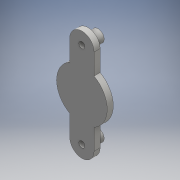
# Autodesk Inventor part: Coperchio Superiore
Saved by Autodesk Inventor 2016 (Build 200138000, 138)
## iProperties
Created: 2016-09-08
Part Number: Coperchio Superiore
Material: Generic
Document SubType Name: Modeling
Designer: Muhammad
Density: 1 g/cm^3
Appearance: Default
Author: Muhammad
Autodesk Inventor part; units mm, degrees
ref_plane "YZ Plane" through (0, 0, 0) normal (1, 0, 0) x (0, 1, 0)
ref_plane "XZ Plane" through (0, 0, 0) normal (0, 1, 0) x (-1, 0, 0)
ref_plane "XY Plane" through (0, 0, 0) normal (0, 0, 1) x (1, 0, 0)
sketch "Sketch1" plane through (0, 0, 0) normal (0, 1, 0) x (-1, 0, 0)
  arc A0 (12, 42.5) -> (-12, 42.5) centre (0, 42.5) ccw
  arc A1 (-12, -42.5) -> (12, -42.5) centre (0, -42.5) ccw
  line L0 (0, 42.5) -> (12, 42.5) construction
  line L1 (0, -42.5) -> (12, -42.5) construction
  line L2 (0, -42.5) -> (-12, -42.5) construction
  line L3 (0, 42.5) -> (-12, 42.5) construction
  line L4 (12, 42.5) -> (12, 21.9317)
  line L5 (12, -42.5) -> (12, -21.9317)
  line L6 (-12, -42.5) -> (-12, -21.9317)
  line L7 (-12, 42.5) -> (-12, 21.9317)
  arc A2 (-12, 21.9317) -> (-12, -21.9317) centre (0, 0) ccw
  arc A3 (12, -21.9317) -> (12, 21.9317) centre (0, 0) ccw
  constraints: 16 end point, 8 point on circle, 4 centre point, 4 point on line, 2 parallel, 1 horizontal, 1 perpendicular, 1 tangent
extrude "Extrusion1" add sketch "Sketch1" along normal blind 6
sketch "Sketch2" plane through (0, 6, 0) normal (0, 1, 0) x (1, 0, 0)
  circle A0 centre (0, 0) radius 10
  circle A1 centre (0, 0) radius 19.5 construction
  arc A2 (-12, -42.5) -> (12, -42.5) centre (0, -42.5) ccw construction
  line L0 (0, -42.5) -> (0, -54.5) construction
  arc A3 (12, 42.5) -> (-12, 42.5) centre (0, 42.5) ccw construction
  line L1 (0, 42.5) -> (0, 54.5) construction
  circle A4 centre (0, -42.5) radius 6
  circle A5 centre (0, -42.5) radius 3
  circle A6 centre (0, 42.5) radius 6
  circle A7 centre (0, 42.5) radius 3
  dimension "d11" = 20
  dimension "d12" = 39
  constraints: 6 centre point, 6 coincident, 4 end point, 2 point on circle, 1 point on line, 1 vertical
  measures "d11" diameter of A0
  measures "d12" diameter of A1
extrude "Extrusion2" add sketch "Sketch2" along normal blind 10 contours A4 | A6
sketch "Sketch3" plane through (0, 6, 42.5) normal (0, 1, 0) x (1, 0, 0)
  circle A0 centre (0, 0) radius 3 projected
  circle A1 centre (0, 0) radius 3
  point P0 (0, 42.5)
  constraints: 1 centre point, 1 coincident
extrude "Extrusion3" cut sketch "Sketch3" against normal blind 7
sketch "Sketch4" plane through (0, 6, -42.5) normal (0, 1, 0) x (1, 0, 0)
  circle A0 centre (0, 0) radius 3
  point P0 (0, -42.5)
  constraints: 1 centre point
extrude "Extrusion4" cut sketch "Sketch4" against normal blind 7
sketch "Sketch5" plane through (0, 6, 0) normal (0, 1, 0) x (1, 0, 0)
  circle A0 centre (0, 0) radius 10
  dimension "d23" = 20
  constraints: 1 centre point, 1 coincident
  measures "d23" diameter of A0
extrude "Extrusion5" add sketch "Sketch5" along normal blind 2
fillet "Fillet1" radius 1.5 1 edges at (-10, 8, 0)
body "Solid1"
